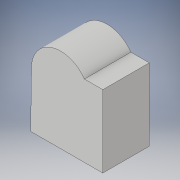
# Autodesk Inventor part: angle
Saved by Autodesk Inventor 2019 (Build 230136000, 136)
## iProperties
Created: 2020-02-20
Part Number: angle
Material: Generic
Document SubType Name: Modeling
Designer: ADMIN
Density: 1 g/cm^3
Appearance: Default
Author: ADMIN
Autodesk Inventor part; units mm, degrees
ref_plane "YZ Plane" through (0, 0, 0) normal (1, 0, 0) x (0, 1, 0)
ref_plane "XZ Plane" through (0, 0, 0) normal (0, 1, 0) x (-1, 0, 0)
ref_plane "XY Plane" through (0, 0, 0) normal (0, 0, 1) x (1, 0, 0)
sketch "Sketch1" plane through (0, 0, 0) normal (0, 0, 1) x (1, 0, 0)
  line L0 (-14.1696, -13.3655) -> (-13.3819, 46.6293)
  line L1 (-13.3819, 46.6293) -> (-13.3819, 46.6293)
  arc A0 (43.6074, 64.3338) -> (-13.3819, 46.6293) centre (17.9908, 46.2174) ccw
  line L2 (43.6074, 64.3338) -> (63.4186, 64.3338)
  line L3 (63.4186, 64.3338) -> (63.4186, -13.3655)
  line L4 (63.4186, -13.3655) -> (-14.1696, -13.3655)
  point P0 (0, 0)
  dimension "d0" = 60
  constraints: 10 end point, 2 perpendicular, 2 point on circle, 1 centre point, 1 horizontal, 1 tangent
  measures "d0" distance of L0.start L0.end
extrude "Extrusion1" add sketch "Sketch1" along normal blind 50
body "Solid1"
